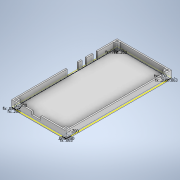
# Autodesk Inventor part: cover_bottom
Saved by Autodesk Inventor 2022 (Build 260153000, 153)
## iProperties
Created: 2022-08-24
Part Number: cover_bottom
Material: Generic
Document SubType Name: Modeling
Designer: suerfu
Density: 1 g/cm^3
Appearance: Default
Author: suerfu
Autodesk Inventor part; units mm, degrees
ref_plane "YZ Plane" through (0, 0, 0) normal (1, 0, 0) x (0, 1, 0)
ref_plane "XZ Plane" through (0, 0, 0) normal (0, 1, 0) x (-1, 0, 0)
ref_plane "XY Plane" through (0, 0, 0) normal (0, 0, 1) x (1, 0, 0)
sketch "Sketch1" plane through (0, 0, 0) normal (0, 1, 0) x (-1, 0, 0)
  line L0 (0, 0) -> (62.23, 0)
  line L1 (62.23, 0) -> (62.23, -120.65)
  line L2 (62.23, -120.65) -> (0, -120.65)
  line L3 (0, -120.65) -> (0, 0)
  dimension "d0" = 62.23
  dimension "d1" = 120.65
  constraints: 8 end point, 2 parallel, 1 horizontal, 1 perpendicular
  measures "d0" distance of L0.start L0.end
  measures "d1" distance of L2.end L0.start
extrude "Extrusion1" add sketch "Sketch1" along normal blind 1.5
sketch "Sketch2" plane through (0, 1.5, 0) normal (0, 1, 0) x (1, 0, 0)
  line L0 (-60.6425, 1.5875) -> (-1.5875, 1.5875)
  line L1 (-1.5875, 1.5875) -> (-1.5875, 119.0625)
  line L2 (-1.5875, 119.0625) -> (-60.6425, 119.0625)
  line L3 (-60.6425, 119.0625) -> (-60.6425, 1.5875)
  line L4 (-62.23, 0) -> (0, 0) projected
  line L5 (0, 0) -> (0, 120.65) projected
  line L6 (-62.23, 120.65) -> (-62.23, 0) projected
  line L7 (0, 120.65) -> (-62.23, 120.65) projected
  line L8 (0, 0) -> (-5.08, 0)
  line L9 (-5.08, 0) -> (-5.08, 5.08)
  line L10 (-5.08, 5.08) -> (0, 5.08)
  line L11 (0, 5.08) -> (0, 0)
  line L12 (-62.23, 0) -> (-57.15, 0)
  line L13 (-57.15, 0) -> (-57.15, 5.08)
  line L14 (-57.15, 5.08) -> (-62.23, 5.08)
  line L15 (-62.23, 5.08) -> (-62.23, 0)
  line L16 (0, 120.65) -> (-5.08, 120.65)
  line L17 (-5.08, 120.65) -> (-5.08, 115.57)
  line L18 (-5.08, 115.57) -> (0, 115.57)
  line L19 (0, 115.57) -> (0, 120.65)
  line L20 (-62.23, 120.65) -> (-57.15, 120.65)
  line L21 (-57.15, 120.65) -> (-57.15, 115.57)
  line L22 (-57.15, 115.57) -> (-62.23, 115.57)
  line L23 (-62.23, 115.57) -> (-62.23, 120.65)
  point P0 (0, 115.57)
  point P1 (-1.5875, 115.57)
  point P2 (-1.5875, 5.08)
  point P3 (-5.08, 1.5875)
  point P4 (-57.15, 1.5875)
  point P5 (-60.6425, 5.08)
  point P6 (-5.08, 119.0625)
  point P7 (-60.6425, 115.57)
  point P8 (-57.15, 119.0625)
  dimension "d4" = 1.5875
  dimension "d5" = 1.5875
  dimension "d6" = 1.5875
  dimension "d7" = 1.5875
  dimension "d8" = 5.08
  dimension "d9" = 5.08
  dimension "d10" = 5.08
  dimension "d11" = 5.08
  dimension "d12" = 5.08
  dimension "d13" = 5.08
  dimension "d14" = 5.08
  dimension "d15" = 5.08
  constraints: 40 end point, 10 parallel, 5 horizontal, 5 perpendicular, 1 collinear, 1 point on line
  measures "d4" distance between parallel lines of L0 L4
  measures "d5" distance between parallel lines of L5 L1
  measures "d6" distance between parallel lines of L6 L3
  measures "d7" distance between parallel lines of L7 L2
  measures "d8" distance of L9.end L10.end
  measures "d9" distance between parallel lines of L4 L10
  measures "d10" distance of L12.end L13.end
  measures "d11" distance of L13.end L14.end
  measures "d12" distance of L21.end L22.end
  measures "d13" distance of L20.end L21.end
  measures "d14" distance of L16.end L17.end
  measures "d15" distance of L17.end L18.end
extrude "Extrusion3" add sketch "Sketch2" along normal blind 7.5 contours L3 L14 L13 L0 | L0 L13 L4 L6 L14 L3 | L0 L9 L4 L13 | L14 L6 L22 L3 | L9 L10 L1 L0 | L0 L1 L10 L5 L4 L9 | L22 L6 L7 L21 L2 L3 | L3 L2 L21 L22 | L1 L18 L5 L10 | L21 L7 L17 L2 | L18 L17 L2 L1 | L1 L2 L17 L7 L5 L18
sketch "Sketch3" plane through (0, 9, 0) normal (0, 1, 0) x (1, 0, 0)
  line L0 (-62.23, 0) -> (0, 0) projected
  line L1 (-39.23, 0) -> (-29, 0)
  line L2 (-29, 0) -> (-29, 1.5875)
  line L3 (-29, 1.5875) -> (-39.23, 1.5875)
  line L4 (-39.23, 1.5875) -> (-39.23, 0)
  line L5 (0, 0) -> (0, 120.65) projected
  line L6 (-62.23, 120.65) -> (-62.23, 0) projected
  line L7 (0, 120.65) -> (-62.23, 120.65) projected
  line L8 (-60.6425, 115.57) -> (-60.6425, 5.08) projected
  line L9 (-62.23, 60.325) -> (-60.6425, 60.325)
  line L10 (-60.6425, 60.325) -> (-60.6425, 98.425)
  line L11 (-60.6425, 98.425) -> (-62.23, 98.425)
  line L12 (-62.23, 98.425) -> (-62.23, 60.325)
  point P0 (-59.69, 2.54)
  point P1 (-59.69, 118.11)
  point P2 (-2.54, 118.11)
  point P3 (-2.54, 2.54)
  dimension "d20" = 29
  dimension "d21" = 23
  dimension "d22" = 2.54
  dimension "d23" = 2.54
  dimension "d24" = 2.54
  dimension "d25" = 2.54
  dimension "d26" = 2.54
  dimension "d27" = 2.54
  dimension "d28" = 2.54
  dimension "d29" = 2.54
  dimension "d47" = 60.325
  dimension "d48" = 22.225
  constraints: 16 end point, 4 parallel, 2 horizontal, 2 perpendicular, 2 point on line, 1 midpoint
  measures "d20" distance between parallel lines of L5 L2
  measures "d21" distance between parallel lines of L6 L4
  measures "d22" distance from line of L0 point (-59.69, 2.54)
  measures "d23" distance from line of L6 point (-59.69, 2.54)
  measures "d24" distance from line of L6 point (-59.69, 118.11)
  measures "d25" distance from line of L7 point (-59.69, 118.11)
  measures "d26" distance from line of L7 point (-2.54, 118.11)
  measures "d27" distance from line of L5 point (-2.54, 118.11)
  measures "d28" distance from line of L5 point (-2.54, 2.54)
  measures "d29" distance from line of L0 point (-2.54, 2.54)
  measures "d47" distance between parallel lines of L0 L9
  measures "d48" distance between parallel lines of L7 L11
extrude "Extrusion4" cut sketch "Sketch3" against normal blind 3.81 contours L4 L3 L2 L0
sketch "Sketch4" plane through (0, 9, 0) normal (0, 1, 0) x (1, 0, 0)
  line L0 (-29, 0) -> (0, 0) projected
  line L1 (0, 0) -> (0, 120.65) projected
  line L2 (-62.23, 0) -> (-39.23, 0) projected
  line L3 (-62.23, 120.65) -> (-62.23, 0) projected
  line L4 (0, 120.65) -> (-62.23, 120.65) projected
  point P0 (-2.54, 2.54)
  point P1 (-2.54, 118.11)
  point P2 (-59.69, 118.11)
  point P3 (-59.69, 2.54)
  dimension "d39" = 2.54
  dimension "d40" = 2.54
  dimension "d41" = 2.54
  dimension "d42" = 2.54
  dimension "d43" = 2.54
  dimension "d44" = 2.54
  dimension "d45" = 2.54
  dimension "d46" = 2.54
  measures "d39" distance from line of L0 point (-2.54, 2.54)
  measures "d40" distance from line of L1 point (-2.54, 2.54)
  measures "d41" distance from line of L2 point (-59.69, 2.54)
  measures "d42" distance from line of L3 point (-59.69, 2.54)
  measures "d43" distance from line of L3 point (-59.69, 118.11)
  measures "d44" distance from line of L4 point (-59.69, 118.11)
  measures "d45" distance from line of L4 point (-2.54, 118.11)
  measures "d46" distance from line of L1 point (-2.54, 118.11)
hole "Hole1" at (-2.54, 9, -2.54) at (-2.54, 9, -118.11) at (-59.69, 9, -118.11) at (-59.69, 9, -2.54) direction (0, -1, 0) diameter 2.4384 depth 5.08 clearance for "Socket Head Cap Screw" size "#2" standard "Ansi Unified Screw Threads"
sketch "Sketch5" plane through (0, 9, 0) normal (0, 1, 0) x (1, 0, 0)
  line L0 (-62.23, 91.65) -> (-60.6425, 91.65)
  line L1 (-60.6425, 5.08) -> (-60.6425, 115.57) projected
  line L2 (-62.23, 120.65) -> (-62.23, 0) projected
  line L3 (-62.23, 79) -> (-60.6425, 79)
  line L4 (-62.23, 84) -> (-60.6425, 84)
  line L5 (-62.23, 75) -> (-60.6425, 75)
  line L6 (-62.23, 62) -> (-60.6425, 62)
  line L7 (-62.23, 0) -> (-39.23, 0) projected
  line L8 (0, 120.65) -> (-62.23, 120.65) projected
  line L9 (-62.23, 96.65) -> (-60.6425, 96.65)
  point P0 (0, 0)
  dimension "d49" = 62
  dimension "d50" = 75
  dimension "d51" = 79
  dimension "d52" = 5
  dimension "d53" = 29
  dimension "d54" = 5
  constraints: 12 end point, 11 point on line, 4 perpendicular, 1 horizontal, 1 parallel
  measures "d49" distance between parallel lines of L7 L6
  measures "d50" distance from line of L7 L5.start
  measures "d51" distance between parallel lines of L7 L3
  measures "d52" distance between parallel lines of L3 L4
  measures "d53" distance between parallel lines of L0 L8
  measures "d54" distance between parallel lines of L0 L9
extrude "Extrusion5" cut sketch "Sketch5" against normal up to surface (7.5 mm away) contours L2 L9 L1 L0 | L4 L1 L3 L2 | L5 L1 L6 L2
equation "\"d4\" = d5"
equation "\"d6\" = d5"
equation "\"d7\" = d5"
equation "\"d10\" = d8"
equation "\"d11\" = d10"
equation "\"d12\" = d8"
equation "\"d13\" = d8"
equation "\"d14\" = d8"
equation "\"d15\" = d8"
equation "\"d24\" = d22"
equation "\"d25\" = d24"
equation "\"d26\" = d25"
equation "\"d27\" = d26"
equation "\"d28\" = d22"
equation "\"d29\" = d28"
equation "\"d40\" = d39"
equation "\"d41\" = d39"
equation "\"d42\" = d41"
equation "\"d43\" = d42"
equation "\"d44\" = d43"
equation "\"d45\" = d44"
equation "\"d46\" = d45"
body "Solid1"
